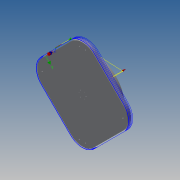
# Autodesk Inventor part: wheel_rim_mold_C
Saved by Autodesk Inventor 2016 (Build 200138000, 138)
## iProperties
Created: 2014-07-30
Part Number: wheel_rim_mold_C
Material: Générique
Document SubType Name: Modeling
Designer: Yann
Density: 1 g/cm^3
Appearance: Par défaut
Author: Yann
Autodesk Inventor part; units mm, degrees
ref_plane "YZ Plane" through (0, 0, 0) normal (1, 0, 0) x (0, 1, 0)
ref_plane "XZ Plane" through (0, 0, 0) normal (0, 1, 0) x (-1, 0, 0)
ref_plane "XY Plane" through (0, 0, 0) normal (0, 0, 1) x (1, 0, 0)
sketch "Esquisse2" plane through (0, 0, 0) normal (1, 0, 0) x (0, 1, 0)
  line L0 (-23.32, 215.2) -> (-23.32, 200.2) projected
  line L1 (-23.32, 200.2) -> (20.32, 200.2) projected
  spline S0 degree 4 poles (20.32, 200.2) (20.32, 180.2) (33.0773, 176.0923) (50, 129.3731) (47.5, 42) (47.5, 32) knots 1 1 1 1 1 2 3 3 3 3 3 projected
  line L2 (47.5, 32) -> (47.5, 0) projected
  line L3 (-23.32, 200.2) -> (-23.32, 0)
  line L4 (-23.32, 0) -> (47.5, 0)
  line L5 (-39.8184, 0) -> (75.6707, 0) projected
  point P0 (0, 0)
  constraints: 4 end point, 1 parallel, 1 perpendicular
revolve "Révolution1" add sketch "Esquisse2" angle 360 about axis through (0, -10, 0) along (0, 1, 0)
sketch "Esquisse3" plane through (0, -23.32, 0) normal (0, -1, 0) x (1, 0, 0)
  circle A0 centre (-254.2, 0) radius 4 projected
  circle A1 centre (254.2, 0) radius 4 projected
  circle A2 centre (-20, -253.412) radius 4 projected
  circle A3 centre (20, -253.412) radius 4 projected
  circle A4 centre (-20, 253.412) radius 4 projected
  circle A5 centre (20, 253.412) radius 4 projected
  circle A6 centre (-22, 0) radius 2.5 projected
  circle A7 centre (-11, 19.0526) radius 2.5 projected
  circle A8 centre (11, 19.0526) radius 2.5 projected
  circle A9 centre (22, 0) radius 2.5 projected
  circle A10 centre (11, -19.0526) radius 2.5 projected
  circle A11 centre (-11, -19.0526) radius 2.5 projected
  line L0 (70.7107, 254.5584) -> (254.5584, 70.7107) projected
  arc A12 (254.5584, -70.7107) -> (254.5584, 70.7107) centre (183.8478, 0) ccw projected
  line L1 (254.5584, -70.7107) -> (70.7107, -254.5584) projected
  arc A13 (-70.7107, -254.5584) -> (70.7107, -254.5584) centre (0, -183.8478) ccw projected
  line L2 (-70.7107, -254.5584) -> (-254.5584, -70.7107) projected
  arc A14 (-254.5584, 70.7107) -> (-254.5584, -70.7107) centre (-183.8478, 0) ccw projected
  line L3 (-254.5584, 70.7107) -> (-70.7107, 254.5584) projected
  arc A15 (70.7107, 254.5584) -> (-70.7107, 254.5584) centre (0, 183.8478) ccw projected
extrude "Extrusion1" add sketch "Esquisse3" along normal blind 23
sketch "Esquisse6" plane through (0, 47.5, 0) normal (0, 1, 0) x (1, 0, 0)
  circle A0 centre (20, -253.412) radius 4 projected
  circle A1 centre (-20, -253.412) radius 4 projected
  circle A2 centre (20, 253.412) radius 4 projected
  circle A3 centre (-20, 253.412) radius 4 projected
  circle A4 centre (254.2, 0) radius 4 projected
  circle A5 centre (-254.2, 0) radius 4 projected
  circle A6 centre (-11, 19.0526) radius 2.5 projected
  circle A7 centre (11, 19.0526) radius 2.5 projected
  circle A8 centre (22, 0) radius 2.5 projected
  circle A9 centre (11, -19.0526) radius 2.5 projected
  circle A10 centre (-11, -19.0526) radius 2.5 projected
  circle A11 centre (-22, 0) radius 2.5 projected
  line L0 (254.5584, -70.7107) -> (70.7107, -254.5584) projected
  arc A12 (-70.7107, -254.5584) -> (70.7107, -254.5584) centre (0, -183.8478) ccw projected
  line L1 (-70.7107, -254.5584) -> (-254.5584, -70.7107) projected
  arc A13 (-254.5584, 70.7107) -> (-254.5584, -70.7107) centre (-183.8478, 0) ccw projected
  line L2 (-254.5584, 70.7107) -> (-70.7107, 254.5584) projected
  arc A14 (70.7107, 254.5584) -> (-70.7107, 254.5584) centre (0, 183.8478) ccw projected
  line L3 (70.7107, 254.5584) -> (254.5584, 70.7107) projected
  arc A15 (254.5584, -70.7107) -> (254.5584, 70.7107) centre (183.8478, 0) ccw projected
  point P0 (0, -32)
extrude "Extrusion3" cut sketch "Esquisse6" against normal blind 35 contours A6 | A7 | A8 | A9 | A10 | A11
